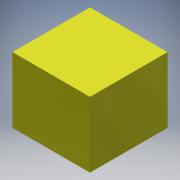
# Autodesk Inventor part: cube
Saved by Autodesk Inventor 2017 SP1 (Build 210196100, 196)
## iProperties
Created: 2018-01-19
Part Number: cube
Material: Generic
Document SubType Name: Modeling
Designer: Ben
Appearance: Smooth - Yellow
Surface Area: 5870.96 cm^2
Volume: 30463.6 cm^3
Author: Ben
Autodesk Inventor part; units mm, degrees
ref_plane "YZ Plane" through (0, 0, 0) normal (1, 0, 0) x (0, 1, 0)
ref_plane "XZ Plane" through (0, 0, 0) normal (0, 1, 0) x (-1, 0, 0)
ref_plane "XY Plane" through (0, 0, 0) normal (0, 0, 1) x (1, 0, 0)
sketch "Sketch1" plane through (0, 0, 0) normal (0, 1, 0) x (-1, 0, 0)
  line L0 (-165.1, 165.1) -> (165.1, 165.1)
  line L1 (165.1, 165.1) -> (165.1, -165.1)
  line L2 (165.1, -165.1) -> (-165.1, -165.1)
  line L3 (-165.1, -165.1) -> (-165.1, 165.1)
  line L4 (-165.1, 165.1) -> (165.1, -165.1) construction
  line L5 (165.1, 165.1) -> (-165.1, -165.1) construction
  point P0 (0, 0)
  dimension "d0" = 330.2
  constraints: 12 end point, 2 midpoint, 2 parallel, 2 perpendicular, 1 horizontal
  measures "d0" distance of L1.end L2.end
extrude "Extrusion1" add sketch "Sketch1" along normal mid plane 279.4
body "Solid1"
